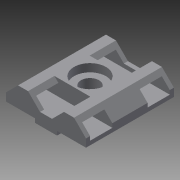
# Autodesk Inventor part: harness clip
Saved by Autodesk Inventor 2015 SP1 (Build 190203100, 203)
## iProperties
Created: 2015-02-19
Part Number: harness clip
Material: Generic
Document SubType Name: Modeling
Designer: Joseph
Density: 1 g/cm^3
Appearance: Default
Author: Joseph
Autodesk Inventor part; units mm, degrees
ref_plane "YZ Plane" through (0, 0, 0) normal (1, 0, 0) x (0, 1, 0)
ref_plane "XZ Plane" through (0, 0, 0) normal (0, 1, 0) x (-1, 0, 0)
ref_plane "XY Plane" through (0, 0, 0) normal (0, 0, 1) x (1, 0, 0)
sketch "Sketch1" plane through (0, 0, 0) normal (0, 0, 1) x (1, 0, 0)
  line L0 (10, 11) -> (-10, 11)
  line L1 (-10, 11) -> (-10, -11)
  line L2 (-10, -11) -> (10, -11)
  line L3 (10, -11) -> (10, 11)
  line L4 (10, 11) -> (-10, -11) construction
  line L5 (-10, 11) -> (10, -11) construction
  line L6 (0, -12.7143) -> (0, 12.7143) construction
  line L7 (12, 0) -> (-13.2325, 0) construction
  point P0 (0, 0)
  dimension "d0" = 20
  dimension "d1" = 22
  constraints: 16 end point, 3 horizontal, 3 midpoint, 2 parallel, 2 vertical, 1 perpendicular, 1 point on line
  measures "d0" distance of L2.end L1.end
  measures "d1" distance of L1.end L0.end
extrude "Extrusion1" add sketch "Sketch1" along normal blind 5
chamfer "Chamfer7" distance 3 angle 45 2 edges at (10, 0, 5) (-10, 0, 5)
sketch "Sketch2" plane through (0, 0, 0) normal (0, 0, -1) x (-1, 0, 0)
  line L0 (2, 1.1547) -> (2, -1.1547) projected
  line L1 (2, -1.1547) -> (0, -2.3094) projected
  line L2 (0, -2.3094) -> (-2, -1.1547) projected
  line L3 (-2, -1.1547) -> (-2, 1.1547) projected
  line L4 (-2, 1.1547) -> (0, 2.3094) projected
  line L5 (0, 2.3094) -> (2, 1.1547) projected
  line L6 (10, -11) -> (-10, -11) projected
  line L7 (-2.75, 11) -> (2.75, 11)
  line L8 (2.75, 11) -> (2.75, -11)
  line L9 (2.75, -11) -> (-2.75, -11)
  line L10 (-2.75, -11) -> (-2.75, 11)
  line L11 (-2.75, 11) -> (2.75, -11) construction
  line L12 (2.75, 11) -> (-2.75, -11) construction
  point P0 (0, 0)
  dimension "d5" = 5.5
  constraints: 12 end point, 2 midpoint, 2 parallel, 1 horizontal, 1 perpendicular, 1 point on line
  measures "d5" distance of L8.end L9.end
extrude "Extrusion2" add sketch "Sketch2" along normal blind 1
sketch "Sketch3" plane through (0, 0, -1) normal (0, 0, -1) x (-1, 0, 0)
  line L0 (2, -1.1547) -> (0, -2.3094) projected
  line L1 (0, -2.3094) -> (-2, -1.1547) projected
  line L2 (-2, -1.1547) -> (-2, 1.1547) projected
  line L3 (-2, 1.1547) -> (0, 2.3094) projected
  line L4 (0, 2.3094) -> (2, 1.1547) projected
  line L5 (2, 1.1547) -> (2, -1.1547) projected
  line L6 (-2.75, 2.75) -> (2.75, 2.75)
  line L7 (2.75, 2.75) -> (2.75, -2.75)
  line L8 (2.75, -2.75) -> (-2.75, -2.75)
  line L9 (-2.75, -2.75) -> (-2.75, 2.75)
  line L10 (-2.75, 2.75) -> (2.75, -2.75) construction
  line L11 (2.75, 2.75) -> (-2.75, -2.75) construction
  point P0 (0, 0)
  dimension "d8" = 5.5
  dimension "d9" = 5.5
  constraints: 12 end point, 2 midpoint, 2 parallel, 1 horizontal, 1 perpendicular
  measures "d8" distance of L7.end L8.end
  measures "d9" distance of L6.end L7.end
extrude "Extrusion3" cut sketch "Sketch3" against normal up to surface (1 mm away) from surface at 0
sketch "Sketch8" plane through (0, 0, 5) normal (0, 0, 1) x (1, 0, 0)
  line L0 (-7, -11) -> (7, -11) projected
  line L1 (7, 11) -> (-7, 11) projected
  line L2 (-1.5, -11) -> (1.5, -11)
  line L3 (1.5, -11) -> (1.5, -4.4105)
  line L4 (1.5, -4.4105) -> (-1.5, -4.4105)
  line L5 (-1.5, -4.4105) -> (-1.5, -11)
  line L6 (-1.5, 11) -> (1.5, 11)
  line L7 (1.5, 11) -> (1.5, 4.4105)
  line L8 (1.5, 4.4105) -> (-1.5, 4.4105)
  line L9 (-1.5, 4.4105) -> (-1.5, 11)
  line L10 (-1.5, -11) -> (-1.5, 11) construction
  line L11 (1.5, -11) -> (1.5, 11) construction
  line L12 (1.5, 4.4105) -> (0, 0) construction
  line L13 (0, 0) -> (-1.5, 4.4105) construction
  line L14 (1.5, -4.4105) -> (0, 0) construction
  line L15 (-1.5, -4.4105) -> (0, 0) construction
  dimension "d83" = 3
  constraints: 28 end point, 10 point on line, 4 parallel, 4 perpendicular, 2 equal length, 2 horizontal, 1 coincident
  measures "d83" distance between parallel lines of L11 L10
extrude "Extrusion7" cut sketch "Sketch8" against normal blind 3
chamfer "Chamfer8" distance 3 angle 45 4 edges at (-1.5, 7.7052, 5) (-1.5, -7.7052, 5) (1.5, -7.7052, 5) (1.5, 7.7052, 5)
sketch "Sketch9" plane through (10, -11, 0) normal (1, 0, 0) x (0, 0, -1)
  line L0 (-2, 0) -> (-2, 22) construction
  line L1 (-1, -1) -> (-1, 22.6316) construction
  line L2 (-1, 1.0298) -> (-4, 1.0298)
  line L3 (-4, 1.0298) -> (-4, 6.5895)
  line L4 (-4, 6.5895) -> (-1, 6.5895)
  line L5 (-1, 6.5895) -> (-1, 1.0298)
  line L6 (-1, 20.9702) -> (-4, 20.9702)
  line L7 (-4, 20.9702) -> (-4, 15.4105)
  line L8 (-4, 15.4105) -> (-1, 15.4105)
  line L9 (-1, 15.4105) -> (-1, 20.9702)
  line L10 (-5, 6.5895) -> (-2, 6.5895) construction
  line L11 (-2, 15.4105) -> (-5, 15.4105) construction
  point P0 (0, 11)
  dimension "d85" = 1
  constraints: 20 end point, 4 parallel, 3 point on line, 2 equal length, 2 horizontal, 2 perpendicular, 1 vertical
  measures "d85" distance between parallel lines of L1 L0
extrude "Extrusion8" cut sketch "Sketch9" against normal through all
sketch "Sketch10" plane through (0, 0, 5) normal (0, 0, 1) x (1, 0, 0)
  point P0 (0, 0)
  point P1 (0, 0)
  constraints: 1 coincident
hole "Hole2" at (0, 0, 5) direction (0, 0, -1) diameter 4.5 end through all counterbore diameter 8 counterbore depth 2 clearance for "Socket Head Cap Screw" size "M4" standard "Ansi Metric M Profile"
body "Solid1"
